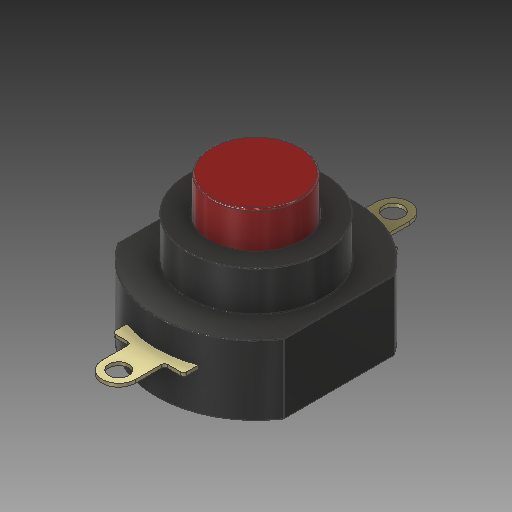
# Autodesk Inventor part: PB-2P-MPBS
Saved by Autodesk Inventor 2018 (Build 220112000, 112)
## iProperties
Created: 2017-10-03
Part Number: PB-2P-MPBS
Material: Generic
Document SubType Name: Modeling
Designer: Rgodino
Density: 1 g/cm^3
Appearance: Plastic Vinyl BLACK
Mass: 0.610481 g
Surface Area: 5.70918 cm^2
Volume: 0.610481 cm^3
Author: Rgodino
Title: Icstation Micro 2 Pin Self Locking SPST Tactile Push Button Switch DC 30V 1A
Autodesk Inventor part; units mm, degrees
ref_plane "YZ Plane" through (0, 0, 0) normal (1, 0, 0) x (0, 1, 0)
ref_plane "XY Plane" through (0, 0, 0) normal (0, 0, 1) x (1, 0, 0)
sketch "Sketch1" plane through (0, 0, 0) normal (0, 1, 0) x (-1, 0, 0)
  line L0 (-5, -3.3166) -> (-5, 3.3166)
  line L1 (5, 3.3166) -> (5, -3.3166)
  line L2 (5, -6) -> (-5, 6) construction
  line L3 (-5, -6) -> (5, 6) construction
  arc A0 (-5, -3.3166) -> (5, -3.3166) centre (0, 0) ccw
  arc A1 (5, 3.3166) -> (-5, 3.3166) centre (0, 0) ccw
  dimension "d3" = 10
  dimension "d4" = 5
  dimension "d5" = 6
  dimension "d6" = 3.3166
  dimension "d7" = 6
  constraints: 8 end point, 4 point on circle, 2 centre point, 2 midpoint, 1 coincident, 1 parallel
  measures "d3" distance between parallel lines of L0 L1
  measures "d4" distance from line of L1 point (0, 0)
  measures "d5" radius of A1
  measures "d6" vertical distance of L1.start point (0, 0)
  measures "d7" radius of A0
extrude "Extrusion1" add sketch "Sketch1" along normal blind 4.2
sketch "Sketch3" plane through (0, 4.2, 0) normal (0, 1, 0) x (1, 0, 0)
  circle A0 centre (0, 0) radius 4.1
  circle A1 centre (0, 0) radius 2.8
  dimension "d26" = 8.2
  dimension "d27" = 5.6
  constraints: 2 centre point, 2 coincident
  measures "d26" diameter of A0
  measures "d27" diameter of A1
extrude "Extrusion3" add sketch "Sketch3" along normal blind 2.4
ref_plane "Work Plane1" through (0, 2.35, 0) normal (0, 1, 0) x (-1, 0, 0)
sketch "Sketch2" plane through (0, 2.35, 0) normal (0, 1, 0) x (-1, 0, 0)
  line L0 (-5, 3.3166) -> (-5, -3.3166) projected
  arc A0 (-5, -3.3166) -> (5, -3.3166) centre (0, 0) ccw projected
  line L1 (5, -3.3166) -> (5, 3.3166) projected
  arc A1 (5, 3.3166) -> (-5, 3.3166) centre (0, 0) ccw projected
  line L2 (-1.2, 6.5) -> (-1.95, 6.5)
  line L3 (-2.15, 6.3) -> (-2.15, -6.3)
  line L4 (-1.95, -6.5) -> (-1.2, -6.5)
  line L5 (2.15, -6.3) -> (2.15, 6.3)
  line L6 (2.15, 6.5) -> (-2.15, -6.5) construction
  line L7 (-2.15, 6.5) -> (2.15, -6.5) construction
  line L8 (0, -9.25) -> (0, -9.25)
  line L9 (0, 9.25) -> (0, 9.25)
  line L10 (1, -9.25) -> (-1, 9.25) construction
  line L11 (-1, -9.25) -> (1, 9.25) construction
  arc A2 (1, 8.25) -> (0, 9.25) centre (0, 8.25) ccw
  arc A3 (0, 9.25) -> (-1, 8.25) centre (0, 8.25) ccw
  arc A4 (-1, -8.25) -> (0, -9.25) centre (0, -8.25) ccw
  arc A5 (0, -9.25) -> (1, -8.25) centre (0, -8.25) ccw
  circle A6 centre (0, 8.25) radius 0.6
  circle A7 centre (0, -8.25) radius 0.6
  line L12 (-1, 6.7) -> (-1, 8.25)
  line L13 (1, 8.25) -> (1, 6.7)
  line L14 (1, -6.7) -> (1, -8.25)
  line L15 (-1, -8.25) -> (-1, -6.7)
  arc A8 (-1.95, 6.5) -> (-2.15, 6.3) centre (-1.95, 6.3) ccw
  arc A9 (-1.2, 6.5) -> (-1, 6.7) centre (-1.2, 6.7) ccw
  arc A10 (-1, -6.7) -> (-1.2, -6.5) centre (-1.2, -6.7) ccw
  line L16 (1.2, -6.5) -> (1.95, -6.5)
  line L17 (1.2, 6.5) -> (1.95, 6.5)
  arc A11 (1, 6.7) -> (1.2, 6.5) centre (1.2, 6.7) ccw
  arc A12 (2.15, 6.3) -> (1.95, 6.5) centre (1.95, 6.3) ccw
  arc A13 (-2.15, -6.3) -> (-1.95, -6.5) centre (-1.95, -6.3) ccw
  arc A14 (1.2, -6.5) -> (1, -6.7) centre (1.2, -6.7) ccw
  arc A15 (1.95, -6.5) -> (2.15, -6.3) centre (1.95, -6.3) ccw
  point P0 (1, 6.5)
  point P1 (1, -6.5)
  dimension "d11" = 4.3
  dimension "d12" = 13
  dimension "d13" = 2
  dimension "d14" = 18.5
  dimension "d15" = 1
  dimension "d16" = 1.2
  dimension "d17" = 1.2
  dimension "d18" = 1.75
  dimension "d19" = 8.25
  dimension "d20" = 1.75
  dimension "d21" = 2
  dimension "d22" = 0.2
  dimension "d23" = 0.2
  constraints: 32 end point, 28 tangent, 24 point on circle, 20 point on line, 14 centre point, 9 equal radius, 8 parallel, 4 midpoint, 3 horizontal, 3 perpendicular, 2 coincident
  measures "d11" distance of L7.end L6.end
  measures "d12" distance of L6.end L7.start
  measures "d13" distance of L10.end L11.end
  measures "d14" distance of L11.start L10.end
  measures "d15" radius of A2
  measures "d16" diameter of A6
  measures "d17" diameter of A7
  measures "d18" distance from line of L4 A5.centre
  measures "d19" distance of A0.centre A4.centre
  measures "d20" distance from line of L2 A3.centre
  measures "d21" distance between parallel lines of L12 L13
  measures "d22" radius of A8
  measures "d23" radius of A11
extrude "Extrusion2" add sketch "Sketch2" along normal blind 0.2 contours L3 A8 L2 A9 L12 A3 A2 L13 A11 L17 A12 L5 A1 | A1 L5 A0 L3 | A0 L5 A15 L16 A14 L14 A5 A4 L15 A10 L4 A13 L3
sketch "Sketch4" plane through (0, 4.2, 0) normal (0, 1, 0) x (1, 0, 0)
  circle A0 centre (0, 0) radius 2.7
  dimension "d30" = 5.4
  constraints: 1 centre point, 1 coincident
  measures "d30" diameter of A0
extrude "Extrusion4" add sketch "Sketch4" along normal blind 4.5
fillet "Fillet1" radius 0.04 15 edges at (5, 4.2, 0) (0, 4.2, 6) (0, 0, 6) (5, 0, 0) (0, 0, -6) (5, 2.1, -3.3166) (5, 2.1, 3.3166) (0, 4.2, -6) (-5, 2.1, 3.3166) (-5, 2.1, -3.3166) (-5, 0, 0) (-5, 4.2, 0) (-4.1, 6.6, 0) (-2.8, 6.6, 0) (-4.1, 4.2, 0)
fillet "Fillet2" radius 0.1 1 edges at (-2.7, 8.7, 0)
equation "\"d17\" = d16"
body "Solid1"
